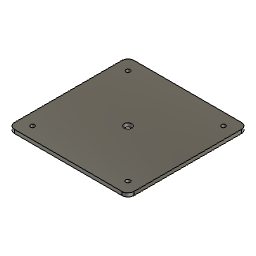
inflow outflow lid v4 (Autodesk Fusion 360 design; units mm, degrees)
Autodesk Fusion 360 part; units mm, degrees
sketch "Sketch1" plane through (0, 0, 0) normal (0, 0, 1) x (1, 0, 0)
  line L0 (0, 0) -> (100, 0)
  line L1 (100, 0) -> (100, 100)
  line L2 (100, 100) -> (0, 100)
  line L3 (0, 100) -> (0, 0)
  dimension "d1" = 100
  dimension "d2" = 100
  constraint horizontal L0
  constraint vertical L1
  constraint horizontal L2
  constraint vertical L3
  constraint coincident L0.start L3.end
  measures "d1" distance of L0.start L0.end
  measures "d2" distance of L0.start L2.end
extrude "Extrude1" add sketch "Sketch1" along normal blind 5
sketch "Sketch2" plane through (0, 0, 5) normal (0, 0, 1) x (-1, 0, 0)
  line L0 (0, -100) -> (0, 0)
  line L1 (0, 0) -> (-100, 0)
  line L2 (-100, 0) -> (-100, -100)
  line L3 (-100, -100) -> (0, -100)
  line L4 (-15, -15) -> (-85, -15)
  line L5 (-85, -15) -> (-85, -85)
  line L6 (-85, -85) -> (-15, -85)
  line L7 (-15, -85) -> (-15, -15)
  line L8 (-15, -85) -> (-10.0503, -89.9497)
  line L9 (-15, -85) -> (-8, -85) construction
  line L10 (-85, -85) -> (-89.9497, -89.9497)
  line L11 (-85, -85) -> (-78, -85) construction
  line L12 (-15, -15) -> (-10.0503, -10.0503)
  line L13 (-15, -15) -> (-8, -15) construction
  line L14 (-85, -15) -> (-89.9497, -10.0503)
  line L15 (-85, -15) -> (-78, -15) construction
  dimension "d5" = 45
  dimension "d6" = 7
  dimension "d7" = 135
  dimension "d8" = 7
  dimension "d9" = 7
  dimension "d10" = 45
  dimension "d11" = 135
  dimension "d12" = 7
  constraint horizontal L4
  constraint vertical L5
  constraint horizontal L6
  constraint vertical L7
  constraint horizontal L9
  constraint horizontal L11
  constraint horizontal L13
  constraint horizontal L15
  measures "d5" angle of L8 L9
  measures "d6" distance of L6.end L8.end
  measures "d7" angle of L10 L11
  measures "d8" distance of L5.end L10.end
  measures "d9" distance of L4.start L12.end
  measures "d10" angle of L12 L13
  measures "d11" angle of L14 L15
  measures "d12" distance of L4.end L14.end
extrude "Extrude2" cut sketch "Sketch2" against normal blind 2 contours L0 L1 L2 L3 | L4 L5 L6 L7
hole "Hole1" at (89.9497, 89.9497, 5) direction (0, 0, -1) diameter 3 depth 67 tip angle 118
hole "Hole2" at (10.0503, 89.9497, 5) direction (0, 0, -1) diameter 3 depth 4.7 tip angle 118
hole "Hole3" at (10.0503, 10.0503, 5) at (89.9497, 10.0503, 5) direction (0, 0, -1) diameter 3 depth 4.7 tip angle 118
hole "Hole4" at (50, 50, 3) direction (0, 0, -1) diameter 6.4 depth 5 tip angle 180
hole "Hole5" at (10.0503, 89.9497, 3) direction (0, 0, -1) diameter 3 depth 5 tip angle 180
hole "Hole6" at (10.0503, 10.0503, 3) direction (0, 0, -1) diameter 3 depth 5 tip angle 180
hole "Hole7" at (89.9497, 10.0503, 3) direction (0, 0, -1) diameter 3 depth 5 tip angle 180
fillet "Fillet1" radius 5 4 edges at (0, 0, 1.5) (100, 0, 1.5) (100, 100, 1.5) (0, 100, 1.5)
hole "Hole8" at (10.0503, 89.9497, 5) at (89.9497, 89.9497, 5) at (10.0503, 10.0503, 5) at (89.9497, 10.0503, 5) direction (0, 0, -1) diameter 3.5 depth 100 tip angle 180
